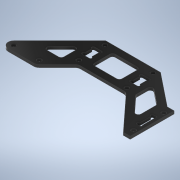
# Autodesk Inventor part: Head_side_frame
Saved by Autodesk Inventor 2020 (Build 240168000, 168)
## iProperties
Part Number: Head_side_frame
Material: GFRP
Document SubType Name: Modeling
Designer: Masato Kubotera
Density: 1.75 g/cm^3
Appearance: 低 光沢 - 黒
Description: GFRP T2
Mass: 6.00647 g
Surface Area: 46.3541 cm^2
Volume: 3.43227 cm^3
Author: Masato Kubotera
Autodesk Inventor part; units mm, degrees
ref_plane "YZ Plane" through (0, 0, 0) normal (1, 0, 0) x (0, 1, 0)
ref_plane "XZ Plane" through (0, 0, 0) normal (0, 1, 0) x (-1, 0, 0)
ref_plane "XY Plane" through (0, 0, 0) normal (0, 0, 1) x (1, 0, 0)
derived "Head_basis.ipt"
sketch "スケッチ1" plane through (0, 0, 0) normal (0, 1, 0) x (-1, 0, 0)
  line L0 (-48.9801, 72.4751) -> (-71.505, 49.9502) construction
  line L1 (4.795, 25.7) -> (-9.205, 25.7)
  line L2 (-2.205, 25.7) -> (-48.9801, 72.4751) construction
  line L3 (-2.205, 25.7) -> (-2.205, 4.9887) construction
  line L4 (-54.888, 55.9606) -> (-58.4235, 59.4962) construction
  line L5 (-58.4235, 59.4962) -> (-81.0509, 36.8688) construction
  line L6 (-81.0509, 36.8688) -> (-77.5154, 33.3332) construction
  line L7 (-77.5154, 33.3332) -> (-54.888, 55.9606) construction
  line L8 (-54.888, 55.9606) -> (-81.0509, 36.8688) construction
  line L9 (-58.4235, 59.4962) -> (-77.5154, 33.3332) construction
  line L10 (-65.9507, 48.4335) -> (-76.5573, 37.8269) construction
  circle A0 centre (-60.1913, 54.1929) radius 1.6
  line L11 (-56.6558, 57.7284) -> (-79.2832, 35.101) construction
  line L12 (17.795, -2.5) -> (-22.205, -2.5) construction
  line L13 (3.8601, -2.5) -> (3.8601, 2.5) construction
  line L14 (5.295, -2.5) -> (5.295, 0)
  line L15 (10.8483, 2.5) -> (7.6861, 2.5)
  line L16 (-9.705, -2.5) -> (-9.705, 0)
  line L17 (5.6869, 2.5) -> (7.6861, 2.5)
  line L18 (-18.705, 0.5) -> (-16.205, 0.5)
  line L19 (-24.705, -2.5) -> (20.295, -2.5)
  arc A1 (5.295, -2.5) -> (7.395, -2.5) centre (6.345, -2.5) ccw
  line L20 (9.935, -2.5) -> (11.935, -2.5)
  line L21 (7.395, -2.5) -> (22.795, -2.5)
  line L22 (22.795, -2.5) -> (22.795, -5.5)
  line L23 (22.795, -5.5) -> (14.045, -5.5)
  line L24 (17.795, -2.5) -> (17.795, -5.5) construction
  arc A2 (-11.805, -2.5) -> (-9.705, -2.5) centre (-10.755, -2.5) ccw
  line L25 (-11.805, -2.5) -> (-27.205, -2.5)
  line L26 (-27.205, -2.5) -> (-27.205, -5.5)
  line L27 (-22.205, -2.5) -> (-22.205, -5.5) construction
  line L28 (-18.455, -5.5) -> (-27.205, -5.5)
  circle A3 centre (-11.5482, -8.5) radius 2
  arc A4 (14.045, -5.5) -> (11.1379, -8.4177) centre (14.045, -8.4071) ccw
  line L29 (15.045, -5.5) -> (15.045, -6.9) construction
  line L30 (15.045, -6.9) -> (20.545, -6.9) construction
  line L31 (20.545, -5.5) -> (20.545, -6.9) construction
  circle A5 centre (-11.5482, -8.5) radius 4
  line L32 (22.795, -2.5) -> (22.795, 0.5)
  line L33 (-2.205, -12.0113) -> (-2.205, 4.9887) construction
  line L34 (-19.455, -5.5) -> (-19.455, -6.9) construction
  line L35 (-19.455, -6.9) -> (-24.955, -6.9) construction
  line L36 (-24.955, -5.5) -> (-24.955, -6.9) construction
  line L37 (-69.7372, 48.1825) -> (-66.2017, 44.6469) construction
  circle A6 centre (-75.7476, 38.6365) radius 1.6
  line L38 (-32.205, -2.5) -> (-22.205, -2.5)
  circle A7 centre (1.665, -21.7132) radius 2
  arc A8 (4.4934, -24.5416) -> (11.1379, -8.4177) centre (-11.5482, -8.5) ccw
  line L39 (-14.3767, -11.3284) -> (-1.1635, -24.5416)
  circle A9 centre (1.665, -21.7132) radius 4
  line L40 (4.4934, -18.8848) -> (-8.7198, -5.6716)
  line L41 (1.665, -21.7132) -> (-11.5482, -8.5) construction
  line L42 (-49.2969, -22.1777) -> (-31.6192, -4.5) construction
  line L43 (-31.6192, -4.5) -> (-28.0837, -8.0355) construction
  line L44 (-28.0837, -8.0355) -> (-45.7614, -25.7132) construction
  line L45 (-45.7614, -25.7132) -> (-49.2969, -22.1777) construction
  line L46 (-49.2969, -22.1777) -> (-28.0837, -8.0355) construction
  line L47 (-31.6192, -4.5) -> (-45.7614, -25.7132) construction
  line L48 (-47.5291, -23.9454) -> (-29.8515, -6.2678) construction
  line L49 (-40.4581, -13.3388) -> (-36.9225, -16.8744) construction
  line L50 (-40.1045, -20.0563) -> (-33.7405, -13.6924) construction
  line L51 (-33.7405, -13.6924) -> (-37.2761, -10.1569) construction
  line L52 (-37.2761, -10.1569) -> (-43.64, -16.5208) construction
  line L53 (-43.64, -16.5208) -> (-40.1045, -20.0563) construction
  line L54 (-40.1045, -20.0563) -> (-37.2761, -10.1569) construction
  line L55 (-33.7405, -13.6924) -> (-43.64, -16.5208) construction
  circle A10 centre (-45.4078, -21.8241) radius 1.6
  line L56 (-42.2258, -15.0359) -> (-38.761, -11.5711)
  line L57 (-37.2761, -10.0861) -> (-33.6698, -13.6924)
  line L58 (-35.1548, -15.1773) -> (-38.6196, -18.6421)
  line L59 (-40.1045, -20.1271) -> (-43.7107, -16.5208)
  line L60 (-43.7107, -16.5208) -> (-33.6698, -13.6924) construction
  line L61 (-37.2761, -10.0861) -> (-40.1045, -20.1271) construction
  arc A11 (-42.2258, -15.0359) -> (-43.7107, -16.5208) centre (-42.9683, -15.7784) ccw
  arc A12 (-37.2761, -10.0861) -> (-38.761, -11.5711) centre (-38.0185, -10.8286) ccw
  circle A13 centre (-31.9728, -8.3891) radius 1.6
  line L62 (-41.8723, -18.2886) -> (-35.5083, -11.9246) construction
  arc A14 (-40.1045, -20.1271) -> (-38.6196, -18.6421) centre (-39.362, -19.3846) ccw
  arc A15 (-35.1548, -15.1773) -> (-33.6698, -13.6924) centre (-34.4123, -14.4349) ccw
  line L63 (-32.205, 17.5) -> (-22.205, 27.5)
  circle A16 centre (-32.205, -2.5) radius 1 construction
  line L64 (-11.5482, -4.5) -> (-31.6192, -4.5)
  line L65 (-58.4235, 59.4962) -> (-54.888, 55.9606)
  line L66 (-77.5154, 33.3332) -> (-81.0509, 36.8688)
  line L67 (-81.0509, 36.8688) -> (-58.4235, 59.4962)
  line L68 (-45.7614, -25.7132) -> (1.665, -25.7132)
  line L69 (-45.7614, -25.7132) -> (-49.2969, -22.1777)
  arc A17 (-15.5479, -8.4464) -> (-18.455, -5.5) centre (-18.455, -8.4074) ccw
  line L70 (-56.368, 20.2487) -> (-52.8324, 16.7132) construction
  line L71 (-52.8324, 16.7132) -> (-70.5101, -0.9645) construction
  line L72 (-56.368, 20.2487) -> (-70.5101, -0.9645) construction
  arc A18 (-66.9746, 9.7128) -> (-68.4595, 8.2279) centre (-67.717, 8.9704) ccw
  line L73 (-59.9035, 9.5714) -> (-63.3683, 6.1066)
  line L74 (-64.8532, 4.6217) -> (-68.4595, 8.2279)
  line L75 (-68.3888, 8.2279) -> (-64.8532, 4.6924) construction
  line L76 (-74.0456, 2.5711) -> (-56.368, 20.2487) construction
  line L77 (-65.2068, 11.4099) -> (-61.6713, 7.8744) construction
  arc A19 (-64.8532, 4.6217) -> (-63.3683, 6.1066) centre (-64.1108, 5.3641) ccw
  line L78 (-66.621, 6.4602) -> (-60.257, 12.8241) construction
  line L79 (-66.9746, 9.7128) -> (-63.5097, 13.1777)
  line L80 (-58.4893, 11.0563) -> (-68.3888, 8.2279) construction
  line L81 (-68.4595, 8.2279) -> (-58.4186, 11.0563) construction
  arc A20 (-59.9035, 9.5714) -> (-58.4186, 11.0563) centre (-59.161, 10.3139) ccw
  line L82 (-64.8532, 4.6924) -> (-58.4893, 11.0563) construction
  line L83 (-62.0248, 14.5919) -> (-68.3888, 8.2279) construction
  arc A21 (-62.0248, 14.6626) -> (-63.5097, 13.1777) centre (-62.7673, 13.9201) ccw
  line L84 (-64.8532, 4.6924) -> (-62.0248, 14.5919) construction
  line L85 (-58.4893, 11.0563) -> (-62.0248, 14.5919) construction
  line L86 (-62.0248, 14.6626) -> (-58.4186, 11.0563)
  circle A22 centre (-56.7215, 16.3597) radius 1.6
  line L87 (-74.0456, 2.5711) -> (-52.8324, 16.7132) construction
  line L88 (-72.2779, 0.8033) -> (-54.6002, 18.481) construction
  line L89 (-62.0248, 14.6626) -> (-64.8532, 4.6217) construction
  line L90 (-70.5101, -0.9645) -> (-74.0456, 2.5711) construction
  circle A23 centre (-70.1565, 2.9246) radius 1.6
  line L91 (-70.5101, -0.9645) -> (-74.0456, 2.5711)
  line L92 (-31.6192, -4.5) -> (-52.8324, 16.7132)
  line L93 (-56.368, 20.2487) -> (-52.8324, 16.7132)
  line L94 (-56.368, 20.2487) -> (-54.888, 55.9606)
  line L95 (-77.5154, 33.3332) -> (-74.0456, 2.5711)
  line L96 (-70.5101, -0.9645) -> (-49.2969, -22.1777)
  line L97 (-54.888, 55.9606) -> (-77.5154, 33.3332) construction
  line L98 (-60.6266, 38.2414) -> (-61.2506, 23.1845)
  line L99 (-61.8347, 21.8531) -> (-67.3045, 16.3833)
  line L100 (-70.7061, 17.5733) -> (-72.169, 30.5433)
  line L101 (-71.5958, 32.1817) -> (-64.0391, 39.7385)
  arc A24 (-60.6266, 38.2414) -> (-64.0391, 39.7385) centre (-62.6249, 38.3243) ccw
  arc A25 (-71.5958, 32.1817) -> (-72.169, 30.5433) centre (-70.1816, 30.7675) ccw
  arc A26 (-70.7061, 17.5733) -> (-67.3045, 16.3833) centre (-68.7187, 17.7975) ccw
  arc A27 (-61.8347, 21.8531) -> (-61.2506, 23.1845) centre (-63.2489, 23.2673) ccw
  line L102 (-15.4772, -17.299) -> (-21.4624, -11.3138)
  line L103 (-24.2908, -11.3138) -> (-30.2761, -17.299)
  line L104 (-28.8619, -20.7132) -> (-16.8914, -20.7132)
  arc A28 (-16.8914, -20.7132) -> (-15.4772, -17.299) centre (-16.8914, -18.7132) ccw
  arc A29 (-21.4624, -11.3138) -> (-24.2908, -11.3138) centre (-22.8766, -12.728) ccw
  arc A30 (-30.2761, -17.299) -> (-28.8619, -20.7132) centre (-28.8619, -18.7132) ccw
  line L105 (-40.1045, -3.0858) -> (-51.4182, 8.2279)
  line L106 (-54.2466, 8.2279) -> (-62.0248, 0.4497)
  line L107 (-62.0248, -2.3787) -> (-50.7111, -13.6924)
  line L108 (-47.8827, -13.6924) -> (-40.1045, -5.9142)
  arc A31 (-40.1045, -5.9142) -> (-40.1045, -3.0858) centre (-41.5187, -4.5) ccw
  arc A32 (-51.4182, 8.2279) -> (-54.2466, 8.2279) centre (-52.8324, 6.8137) ccw
  arc A33 (-62.0248, 0.4497) -> (-62.0248, -2.3787) centre (-60.6106, -0.9645) ccw
  arc A34 (-50.7111, -13.6924) -> (-47.8827, -13.6924) centre (-49.2969, -12.2782) ccw
  circle A35 centre (-11.5482, -8.5) radius 1.6
  circle A36 centre (1.665, -21.7132) radius 1.6
  line L109 (-61.9591, 48.8896) -> (-70.4443, 40.4043) construction
  line L110 (-70.4443, 40.4043) -> (-72.2121, 42.1721) construction
  line L111 (-72.2121, 42.1721) -> (-63.7268, 50.6573) construction
  line L112 (-63.7268, 50.6573) -> (-61.9591, 48.8896) construction
  line L113 (-61.9591, 48.8896) -> (-72.2121, 42.1721) construction
  line L114 (-70.4443, 40.4043) -> (-63.7268, 50.6573) construction
  line L115 (-62.8429, 49.7735) -> (-71.3282, 41.2882) construction
  line L116 (-61.8884, 48.8896) -> (-63.7268, 50.728)
  line L117 (-63.7268, 50.728) -> (-72.2828, 42.1721)
  line L118 (-72.2828, 42.1721) -> (-70.4443, 40.3336)
  line L119 (-70.4443, 40.3336) -> (-61.8884, 48.8896)
  line L120 (-61.8884, 48.8896) -> (-72.2828, 42.1721) construction
  line L121 (-63.7268, 50.728) -> (-70.4443, 40.3336) construction
  arc A37 (-63.3733, 47.4046) -> (-61.8884, 48.8896) centre (-62.6308, 48.1471) ccw
  arc A38 (-62.6768, 49.678) -> (-64.7768, 49.678) centre (-63.7268, 49.678) ccw
  arc A39 (-70.4443, 40.3336) -> (-68.9594, 41.8185) centre (-69.7019, 41.076) ccw
  arc A40 (-71.2328, 43.2221) -> (-71.2328, 41.1221) centre (-71.2328, 42.1721) ccw
  line L122 (-9.705, 0) -> (5.295, 0)
  line L123 (-8.2701, 0) -> (3.8601, 0)
  line L124 (-16.205, 2.5) -> (11.795, 2.5)
  line L125 (-2.205, 2.5) -> (-60.5801, 60.8751) construction
  point P0 (0, 0)
  point P1 (-67.9695, 46.4147)
  point P2 (-14.345, -2.5)
  point P3 (-38.6903, -15.1066)
  point P4 (-38.6903, -15.1066)
  point P5 (-63.439, 9.6421)
  point P6 (-63.439, 9.6421)
  point P7 (-61.2829, 22.4049)
  point P8 (-67.0856, 45.5308)
  point P9 (-67.0856, 45.5308)
  point P10 (-71.2328, 41.1221)
  point P11 (-68.9594, 41.8185)
  dimension "d5" = 0
  measures "d5" distance between parallel lines of L67 L5
extrude "押し出し1" add sketch "スケッチ1" along normal blind 2 contours L64 A5 A17 L28 L26 | L26 L28 A17 A5 L39 A9 L68 L69 L96 L91 L95 L66 L67 L65 L94 L93 L92 L64 | A5 | L40 A9 L39 A5 | A9 | A3 | A7
fillet "フィレット1" radius 4 2 edges at (31.6192, 1, -4.5) (56.368, 1, 20.2487)
